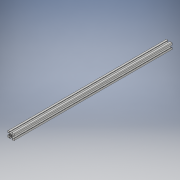
# Autodesk Inventor part: 20-2020-500-CL
Saved by Autodesk Inventor 2025 (Build 290162000, 162)
## iProperties
Created: 2024-07-05
Part Number: 20-2020-500-CL
Material: Generic
Catalog Web Link: www.cadenas.de
Description: 20-2020, 2020-Black-T-Slotted Profile - 20 Series
Vendor: 8020
Document SubType Name: Modeling
Designer: psAdmin
Manufacturer: 8020
Mass: 79.6867 g
Surface Area: 910.39 cm^2
Volume: 79.6867 cm^3
Density: 1 g/cm^3
Appearance: PSOLRGB-191-191-191
Category: PARTsolutions
Company: 8020
PSOL_IDENT_0: {$CADENAS_DATA/23d-libs/8020/metric/profiles/20_series/20_2020.prj},187 {VTYP=3D},{NB=20-2020-500-CL
PSOL_IDENT_1: },{LINA=20-2020-500},{NN=20-2020, 2020-Black},{DATE=01.08.2023 13:37:04},{GEOMDATE=09.02.2018 09:13:
PSOL_IDENT_2: 03},{VERSION=},{LINEID=10},{WBVAR=FIN,LS,L},{WBNUMERIC=L}  {NB=20-2020-500-CL},{LINA=20-2020-500},{K
PSOL_IDENT_3: T=DUMMY},{PN=20-2020-500},{PN1=20-2020},{FIN=CA},{LS=-CL},{L=500.00},{SERIES=20-2020},{MAT=6105-T5 A
PSOL_IDENT_4: luminum},{W=0.4732},{LALG=[25:6000/0.05]},{MIX=0.6826},{MIY=0.6826},{EA=1.5890},{COLOR=.75,.75,.75}
NB: 20-2020-500-CL
NN: 20-2020, 2020-Black
NT: T-Slotted Profile - 20 Series
NBSYN: $PN.$LS.
LINA: 20-2020-500
CATALOG: 80/20
PN: 20-2020-500
FIN: Clear Anodize
LS: Custom Length
L: 500
SERIES: 20-2020
MAT: 6105-T5 Aluminum
W: 0.4732
MIX: 0.6826
MIY: 0.6826
EA: 1.5890
SUPPLIER: 8020
ARTICLENO: 20-2020-500-CL
BOMINFO: 20-2020-500
CREATOR: CADENAS GmbH
Title: 20-2020-500
Author: Cadenas PARTsolutions
Comments: T-Slotted Profile - 20 Series
Autodesk Inventor part; units mm, degrees
ref_plane "YZ Plane" through (0, 0, 0) normal (1, 0, 0) x (0, 1, 0)
ref_plane "XZ Plane" through (0, 0, 0) normal (0, 1, 0) x (-1, 0, 0)
ref_plane "XY Plane" through (0, 0, 0) normal (0, 0, 1) x (1, 0, 0)
sketch "Sketch_1" plane through (0, 0, 0) normal (0, 0, 1) x (1, 0, 0)
  arc A0 (-10, -8.5) -> (-8.5, -10) centre (-8.5, -8.5) ccw
  line L0 (-8.5, -10) -> (-3.138, -10)
  arc A1 (-3.138, -10) -> (-2.63, -9.492) centre (-3.138, -9.492) ccw
  line L1 (-2.63, -9.492) -> (-2.63, -9.008)
  arc A2 (-2.63, -9.008) -> (-3.138, -8.5) centre (-3.138, -9.008) ccw
  line L2 (-3.138, -8.5) -> (-5.487, -8.5)
  arc A3 (-5.995, -7.992) -> (-5.487, -8.5) centre (-5.487, -7.992) ccw
  line L3 (-5.995, -7.992) -> (-5.995, -7.2662)
  arc A4 (-5.8462, -6.907) -> (-5.995, -7.2662) centre (-5.487, -7.2662) ccw
  line L4 (-5.8462, -6.907) -> (-2.743, -3.8038)
  arc A5 (-2.3838, -3.655) -> (-2.743, -3.8038) centre (-2.3838, -4.163) ccw
  line L5 (-2.3838, -3.655) -> (2.3841, -3.655)
  arc A6 (2.7433, -3.8038) -> (2.3841, -3.655) centre (2.3841, -4.163) ccw
  line L6 (2.7433, -3.8038) -> (5.8462, -6.9067)
  arc A7 (5.995, -7.2659) -> (5.8462, -6.9067) centre (5.487, -7.2659) ccw
  line L7 (5.995, -7.2659) -> (5.995, -7.992)
  arc A8 (5.487, -8.5) -> (5.995, -7.992) centre (5.487, -7.992) ccw
  line L8 (5.487, -8.5) -> (3.138, -8.5)
  arc A9 (3.138, -8.5) -> (2.63, -9.008) centre (3.138, -9.008) ccw
  line L9 (2.63, -9.008) -> (2.63, -9.492)
  arc A10 (2.63, -9.492) -> (3.138, -10) centre (3.138, -9.492) ccw
  line L10 (3.138, -10) -> (8.5, -10)
  arc A11 (8.5, -10) -> (10, -8.5) centre (8.5, -8.5) ccw
  line L11 (10, -8.5) -> (10, -3.138)
  arc A12 (10, -3.138) -> (9.492, -2.63) centre (9.492, -3.138) ccw
  line L12 (9.492, -2.63) -> (9.008, -2.63)
  arc A13 (9.008, -2.63) -> (8.5, -3.138) centre (9.008, -3.138) ccw
  line L13 (8.5, -3.138) -> (8.5, -5.487)
  arc A14 (7.992, -5.995) -> (8.5, -5.487) centre (7.992, -5.487) ccw
  line L14 (7.992, -5.995) -> (7.2662, -5.995)
  arc A15 (6.907, -5.8462) -> (7.2662, -5.995) centre (7.2662, -5.487) ccw
  line L15 (6.907, -5.8462) -> (3.8038, -2.743)
  arc A16 (3.655, -2.3838) -> (3.8038, -2.743) centre (4.163, -2.3838) ccw
  line L16 (3.655, -2.3838) -> (3.655, 2.3841)
  arc A17 (3.8038, 2.7433) -> (3.655, 2.3841) centre (4.163, 2.3841) ccw
  line L17 (3.8038, 2.7433) -> (6.9067, 5.8462)
  arc A18 (7.2659, 5.995) -> (6.9067, 5.8462) centre (7.2659, 5.487) ccw
  line L18 (7.2659, 5.995) -> (7.992, 5.995)
  arc A19 (8.5, 5.487) -> (7.992, 5.995) centre (7.992, 5.487) ccw
  line L19 (8.5, 5.487) -> (8.5, 3.138)
  arc A20 (8.5, 3.138) -> (9.008, 2.63) centre (9.008, 3.138) ccw
  line L20 (9.008, 2.63) -> (9.492, 2.63)
  arc A21 (9.492, 2.63) -> (10, 3.138) centre (9.492, 3.138) ccw
  line L21 (10, 3.138) -> (10, 8.5)
  arc A22 (10, 8.5) -> (8.5, 10) centre (8.5, 8.5) ccw
  line L22 (8.5, 10) -> (3.138, 10)
  arc A23 (3.138, 10) -> (2.63, 9.492) centre (3.138, 9.492) ccw
  line L23 (2.63, 9.492) -> (2.63, 9.008)
  arc A24 (2.63, 9.008) -> (3.138, 8.5) centre (3.138, 9.008) ccw
  line L24 (3.138, 8.5) -> (5.487, 8.5)
  arc A25 (5.995, 7.992) -> (5.487, 8.5) centre (5.487, 7.992) ccw
  line L25 (5.995, 7.992) -> (5.995, 7.2662)
  arc A26 (5.8462, 6.907) -> (5.995, 7.2662) centre (5.487, 7.2662) ccw
  line L26 (5.8462, 6.907) -> (2.743, 3.8038)
  arc A27 (2.3838, 3.655) -> (2.743, 3.8038) centre (2.3838, 4.163) ccw
  line L27 (2.3838, 3.655) -> (-2.3841, 3.655)
  arc A28 (-2.7433, 3.8038) -> (-2.3841, 3.655) centre (-2.3841, 4.163) ccw
  line L28 (-2.7433, 3.8038) -> (-5.8462, 6.9067)
  arc A29 (-5.995, 7.2659) -> (-5.8462, 6.9067) centre (-5.487, 7.2659) ccw
  line L29 (-5.995, 7.2659) -> (-5.995, 7.992)
  arc A30 (-5.487, 8.5) -> (-5.995, 7.992) centre (-5.487, 7.992) ccw
  line L30 (-5.487, 8.5) -> (-3.138, 8.5)
  arc A31 (-3.138, 8.5) -> (-2.63, 9.008) centre (-3.138, 9.008) ccw
  line L31 (-2.63, 9.008) -> (-2.63, 9.492)
  arc A32 (-2.63, 9.492) -> (-3.138, 10) centre (-3.138, 9.492) ccw
  line L32 (-3.138, 10) -> (-8.5, 10)
  arc A33 (-8.5, 10) -> (-10, 8.5) centre (-8.5, 8.5) ccw
  line L33 (-10, 8.5) -> (-10, 3.138)
  arc A34 (-10, 3.138) -> (-9.492, 2.63) centre (-9.492, 3.138) ccw
  line L34 (-9.492, 2.63) -> (-9.008, 2.63)
  arc A35 (-9.008, 2.63) -> (-8.5, 3.138) centre (-9.008, 3.138) ccw
  line L35 (-8.5, 3.138) -> (-8.5, 5.487)
  arc A36 (-7.992, 5.995) -> (-8.5, 5.487) centre (-7.992, 5.487) ccw
  line L36 (-7.992, 5.995) -> (-7.2662, 5.995)
  arc A37 (-6.907, 5.8462) -> (-7.2662, 5.995) centre (-7.2662, 5.487) ccw
  line L37 (-6.907, 5.8462) -> (-3.8038, 2.743)
  arc A38 (-3.655, 2.3838) -> (-3.8038, 2.743) centre (-4.163, 2.3838) ccw
  line L38 (-3.655, 2.3838) -> (-3.655, -2.3841)
  arc A39 (-3.8038, -2.7433) -> (-3.655, -2.3841) centre (-4.163, -2.3841) ccw
  line L39 (-3.8038, -2.7433) -> (-6.9067, -5.8462)
  arc A40 (-7.2659, -5.995) -> (-6.9067, -5.8462) centre (-7.2659, -5.487) ccw
  line L40 (-7.2659, -5.995) -> (-7.992, -5.995)
  arc A41 (-8.5, -5.487) -> (-7.992, -5.995) centre (-7.992, -5.487) ccw
  line L41 (-8.5, -5.487) -> (-8.5, -3.138)
  arc A42 (-8.5, -3.138) -> (-9.008, -2.63) centre (-9.008, -3.138) ccw
  line L42 (-9.008, -2.63) -> (-9.492, -2.63)
  arc A43 (-9.492, -2.63) -> (-10, -3.138) centre (-9.492, -3.138) ccw
  line L43 (-10, -3.138) -> (-10, -8.5)
  arc A44 (-1.9358, -0.8037) -> (-2.3045, -2.1245) centre (-1.748, -1.568) ccw
  line L44 (-2.3045, -2.1245) -> (-2.1245, -2.3045)
  arc A45 (-2.1245, -2.3045) -> (-0.8037, -1.9358) centre (-1.568, -1.748) ccw
  arc A46 (-0.8037, -1.9358) -> (0.8037, -1.9358) centre (0, 0) ccw
  arc A47 (0.8037, -1.9358) -> (2.1245, -2.3045) centre (1.568, -1.748) ccw
  line L45 (2.1245, -2.3045) -> (2.3045, -2.1245)
  arc A48 (2.3045, -2.1245) -> (1.9358, -0.8037) centre (1.748, -1.568) ccw
  arc A49 (1.9358, -0.8037) -> (1.9358, 0.8037) centre (0, 0) ccw
  arc A50 (1.9358, 0.8037) -> (2.3045, 2.1245) centre (1.748, 1.568) ccw
  line L46 (2.3045, 2.1245) -> (2.1245, 2.3045)
  arc A51 (2.1245, 2.3045) -> (0.8037, 1.9358) centre (1.568, 1.748) ccw
  arc A52 (0.8037, 1.9358) -> (-0.8037, 1.9358) centre (0, 0) ccw
  arc A53 (-0.8037, 1.9358) -> (-2.1245, 2.3045) centre (-1.568, 1.748) ccw
  line L47 (-2.1245, 2.3045) -> (-2.3045, 2.1245)
  arc A54 (-2.3045, 2.1245) -> (-1.9358, 0.8037) centre (-1.748, 1.568) ccw
  arc A55 (-1.9358, 0.8037) -> (-1.9358, -0.8037) centre (0, 0) ccw
  constraints: 112 point on circle, 96 end point, 56 centre point
extrude "Extrusion1" add sketch "Sketch_1" against normal blind 500
body "Solid1"
